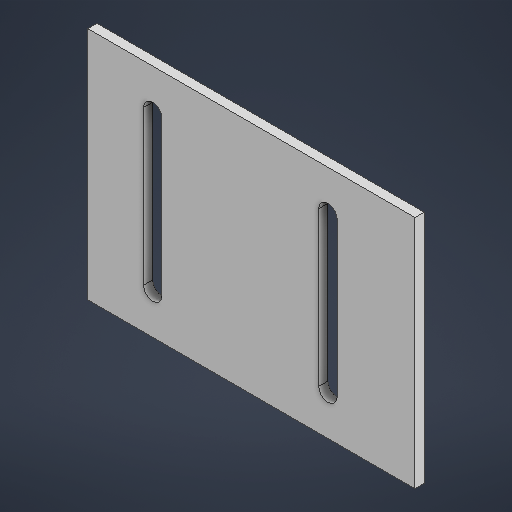
# Autodesk Inventor part: 零件1
Saved by Autodesk Inventor 2025 (Build 290162000, 162)
## iProperties
Created: 2025-11-29
Part Number: 零件1
Material: 常规
Document SubType Name: Modeling
Designer: XH
Density: 1 g/cm^3
Appearance: 默认
Author: XH
Autodesk Inventor part; units mm, degrees
ref_plane "YZ Plane" through (0, 0, 0) normal (1, 0, 0) x (0, 1, 0)
ref_plane "XZ Plane" through (0, 0, 0) normal (0, 1, 0) x (-1, 0, 0)
ref_plane "XY Plane" through (0, 0, 0) normal (0, 0, 1) x (1, 0, 0)
sketch "草图1" plane through (0, 0, 0) normal (0, 0, 1) x (1, 0, 0)
  line L0 (53.15, -38.15) -> (-53.15, -38.15)
  line L1 (-53.15, -38.15) -> (-53.15, 38.15)
  line L2 (-53.15, 38.15) -> (53.15, 38.15)
  line L3 (53.15, 38.15) -> (53.15, -38.15)
  line L4 (53.15, -38.15) -> (-53.15, 38.15) construction
  line L5 (-53.15, -38.15) -> (53.15, 38.15) construction
  point P0 (0, 0)
  dimension "d0" = 106.3
  dimension "d1" = 76.3
  constraints: 12 end point, 2 midpoint, 2 parallel, 1 horizontal, 1 perpendicular
  measures "d0" distance of L1.end L2.end
  measures "d1" distance of L2.end L0.start
extrude "拉伸1" add sketch "草图1" along normal blind 3
sketch "草图4" plane through (0, 0, 3) normal (0, 0, 1) x (1, 0, 0)
  line L0 (24.8622, 25) -> (24.8622, -25) construction
  line L1 (21.8622, 25) -> (21.8622, -25)
  line L2 (27.8622, -25) -> (27.8622, 25)
  arc A0 (27.8622, 25) -> (21.8622, 25) centre (24.8622, 25) ccw
  arc A1 (21.8622, -25) -> (27.8622, -25) centre (24.8622, -25) ccw
  line L3 (-32.0429, 25) -> (-32.0429, -25) construction
  line L4 (-35.0429, 25) -> (-35.0429, -25)
  line L5 (-29.0429, -25) -> (-29.0429, 25)
  arc A2 (-29.0429, 25) -> (-35.0429, 25) centre (-32.0429, 25) ccw
  arc A3 (-35.0429, -25) -> (-29.0429, -25) centre (-32.0429, -25) ccw
  point P0 (0, 0)
  point P1 (24.8622, 0)
  point P2 (-32.0429, 0)
  dimension "d4" = 50
  dimension "d5" = 6
  dimension "d6" = 50
  dimension "d7" = 6
  constraints: 16 end point, 8 point on circle, 8 tangent, 4 centre point, 2 midpoint, 2 parallel, 2 vertical
  measures "d4" distance of L0.start L0.end
  measures "d5" distance between parallel lines of L1 L2
  measures "d6" distance of L3.start L3.end
  measures "d7" distance between parallel lines of L4 L5
extrude "拉伸2" cut sketch "草图4" against normal blind 3
